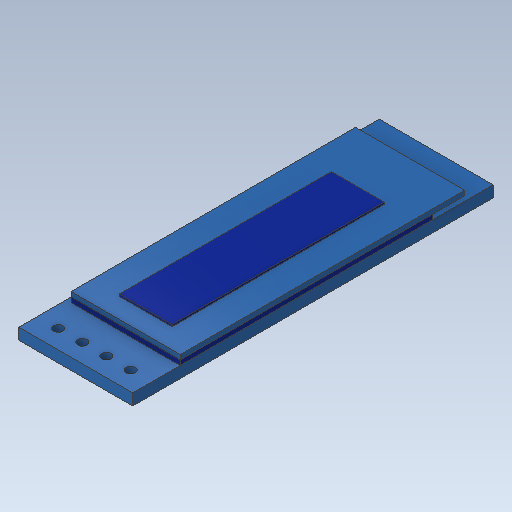
# Autodesk Inventor part: LED Screen 0.91 inch
Saved by Autodesk Inventor 2020.1 (Build 241239000, 239)
## iProperties
Created: 2019-07-16
Part Number: LED Screen 0.91 inch
Material: Generic
Document SubType Name: Modeling
Designer: Petar
Density: 1 g/cm^3
Appearance: Default
Mass: 0.805202 g
Surface Area: 16.0321 cm^2
Volume: 0.805202 cm^3
Author: Petar
Autodesk Inventor part; units mm, degrees
ref_plane "YZ Plane" through (0, 0, 0) normal (1, 0, 0) x (0, 1, 0)
ref_plane "XZ Plane" through (0, 0, 0) normal (0, 1, 0) x (-1, 0, 0)
sketch "Sketch1" plane through (0, 0, 0) normal (0, 1, 0) x (-1, 0, 0)
  line L0 (-6, 19) -> (6, 19)
  line L1 (6, 19) -> (6, -19)
  line L2 (6, -19) -> (-6, -19)
  line L3 (-6, -19) -> (-6, 19)
  line L4 (-6, 19) -> (6, -19) construction
  line L5 (6, 19) -> (-6, -19) construction
  line L6 (5.502, -16) -> (-5.998, -16)
  line L7 (5.502, 14) -> (5.502, -16)
  line L8 (0, 19) -> (0, -19) construction
  line L9 (5.503, 14.001) -> (-5.999, 14.001)
  line L10 (-5.999, 14.001) -> (-5.999, -12.599)
  line L11 (-5.999, -12.599) -> (5.503, -12.599)
  line L12 (3.541, 12.89) -> (-4.039, 12.89)
  line L13 (-4.039, 12.89) -> (-4.039, -11.49)
  line L14 (-4.039, -11.49) -> (3.541, -11.49)
  line L15 (3.541, -11.49) -> (3.541, 12.89)
  line L16 (2.541, 11.89) -> (-3.039, 11.89)
  line L17 (-3.039, 11.89) -> (-3.039, -10.49)
  line L18 (-3.039, -10.49) -> (2.541, -10.49)
  line L19 (2.541, -10.49) -> (2.541, 11.89)
  line L20 (-0.249, 12.89) -> (-0.249, -11.49) construction
  line L21 (3.541, 0.7) -> (-4.039, 0.7) construction
  circle A0 centre (-3.81, 17.04) radius 0.5
  circle A1 centre (-1.27, 17.04) radius 0.5
  circle A2 centre (1.27, 17.04) radius 0.5
  circle A3 centre (3.81, 17.04) radius 0.5
  line L22 (3.041, -13.8) -> (-3.539, -13.8)
  line L23 (-3.539, -13.8) -> (-3.539, -14.8)
  line L24 (-3.539, -14.8) -> (3.041, -14.8)
  line L25 (3.041, -14.8) -> (3.041, -13.8)
  line L26 (5.502, 14) -> (-5.998, 14)
  line L27 (5.503, -12.599) -> (5.503, 14.001)
  line L28 (-5.998, 14) -> (-5.998, -16)
  point P0 (0, 0)
  dimension "d0" = 12
  dimension "d1" = 38
  dimension "d2" = 3
  dimension "d3" = 30
  dimension "d5" = 26.6
  dimension "d6" = 7.58
  dimension "d7" = 24.38
  dimension "d8" = 5.58
  dimension "d9" = 22.38
  dimension "d10" = 1.96
  dimension "d11" = 7.51
  dimension "d13" = 2.19
  dimension "d14" = 1.96
  dimension "d15" = 1
  dimension "d18" = 2.54
  dimension "d27" = 1
  dimension "d28" = 1.2
  dimension "d32" = 0.001
  dimension "d33" = 0.001
  dimension "d34" = 0.001
  dimension "d35" = 11.5
  dimension "d36" = 0.001
  constraints: 58 end point, 11 parallel, 8 midpoint, 7 horizontal, 5 perpendicular, 4 centre point, 1 vertical, 10 other
  measures "d0" distance of L1.end L2.end
  measures "d1" distance of L0.end L1.end
  measures "d2" distance between parallel lines of L2 L6
  measures "d3" distance of L7.start L6.start
  measures "d5" distance of L10.end L9.end
  measures "d6" distance of L14.end L13.end
  measures "d7" distance of L13.end L12.end
  measures "d8" distance of L18.end L17.end
  measures "d9" distance of L17.end L16.end
  measures "d10" distance between parallel lines of L10 L13
  measures "d11" distance between parallel lines of L14 L2
  measures "d13" distance from line of L3 A0.centre
  measures "d14" distance from line of L0 A0.centre
  measures "d15" diameter of A0
  measures "d18" distance of A0.centre A1.centre
  measures "d27" distance of L23.end L22.end
  measures "d28" distance between parallel lines of L6 L24
  measures "d32" distance between parallel lines of L7 L27
  measures "d33" distance between parallel lines of L3 L10
  measures "d34" distance between parallel lines of L10 L28
  measures "d35" distance between parallel lines of L28 L7
  measures "d36" distance between parallel lines of L26 L9
extrude "Extrusion1" add sketch "Sketch1" against normal blind 1.2 contours L0 L1 L2 L3 L6 L7 L9 | L9 L7 L11 L3 | L11 L7 L6 L3 | L15 L14 L13 L12 | L19 L18 L17 L16 | L25 L24 L23 L22
extrude "Extrusion2" add sketch "Sketch1" along normal blind 0.5 contours L9 L7 L11 L3 | L15 L14 L13 L12 | L19 L18 L17 L16 | L25 L24 L23 L22
sketch "Sketch2" plane through (0, 0.5, 0) normal (0, 1, 0) x (1, 0, 0)
  line L0 (-5.502, -14) -> (-5.502, 16) projected
  line L1 (-5.502, 16) -> (5.998, 16) projected
  line L2 (-5.502, -14) -> (5.998, -14) projected
  line L3 (5.998, -14) -> (5.998, 16) projected
  line L4 (-3.541, -12.89) -> (4.039, -12.89) projected
  line L5 (-3.541, 11.49) -> (-3.541, -12.89) projected
  line L6 (4.039, -12.89) -> (4.039, 11.49) projected
  line L7 (4.039, 11.49) -> (-3.541, 11.49) projected
  point P0 (0, 0)
extrude "Extrusion3" add sketch "Sketch2" along normal blind 0.5 contours L0 L1 L3 L2 | L5 L7 L6 L4
sketch "Sketch3" plane through (0, 1, 0) normal (0, 1, 0) x (1, 0, 0)
  line L0 (-2.541, -11.89) -> (3.039, -11.89) projected
  line L1 (-2.541, 10.49) -> (-2.541, -11.89) projected
  line L2 (3.039, -11.89) -> (3.039, 10.49) projected
  line L3 (3.039, 10.49) -> (-2.541, 10.49) projected
  point P0 (0, 0)
extrude "Extrusion4" add sketch "Sketch3" along normal blind 0.2
extrude "Extrusion5" cut sketch "Sketch2" against normal blind 0.5 contours L5 L7 L6 L4
fillet "Fillet1" radius 1 4 edges at (-3.541, 0.25, 12.89) (4.039, 0.25, -11.49) (-3.541, 0.25, -11.49) (4.039, 0.25, 12.89)
sketch "Sketch4" plane through (0, -1.2, 0) normal (0, 1, 0) x (1, 0, 0)
  line L0 (2.785, -15.895) -> (2.585, -16.095)
  line L1 (2.585, -16.095) -> (2.585, -17.985)
  line L2 (2.585, -17.985) -> (2.785, -18.185)
  line L3 (2.785, -18.185) -> (4.835, -18.185)
  line L4 (4.835, -18.185) -> (5.035, -17.985)
  line L5 (5.035, -17.985) -> (5.035, -16.095)
  line L6 (5.035, -16.095) -> (4.835, -15.895)
  line L7 (4.835, -15.895) -> (2.785, -15.895)
  line L8 (3.81, -18.185) -> (3.81, -15.895) construction
  line L9 (2.585, -17.04) -> (5.035, -17.04) construction
  circle A0 centre (3.81, -17.04) radius 0.5 construction
  line L10 (3.51, -17.34) -> (4.11, -17.34)
  line L11 (4.11, -17.34) -> (4.11, -16.74)
  line L12 (4.11, -16.74) -> (3.51, -16.74)
  line L13 (3.51, -16.74) -> (3.51, -17.34)
  line L14 (3.51, -17.34) -> (4.11, -16.74) construction
  line L15 (4.11, -17.34) -> (3.51, -16.74) construction
  line L16 (6, -19) -> (-6, -19) construction
  line L17 (0.245, -15.895) -> (0.045, -16.095)
  line L18 (0.045, -16.095) -> (0.045, -17.985)
  line L19 (0.045, -17.985) -> (0.245, -18.185)
  line L20 (0.245, -18.185) -> (2.295, -18.185)
  line L21 (2.295, -18.185) -> (2.495, -17.985)
  line L22 (2.495, -17.985) -> (2.495, -16.095)
  line L23 (2.495, -16.095) -> (2.295, -15.895)
  line L24 (2.295, -15.895) -> (0.245, -15.895)
  line L25 (1.27, -18.185) -> (1.27, -15.895) construction
  line L26 (0.045, -17.04) -> (2.495, -17.04) construction
  circle A1 centre (1.27, -17.04) radius 0.5 construction
  line L27 (0.97, -17.34) -> (1.57, -17.34)
  line L28 (1.57, -17.34) -> (1.57, -16.74)
  line L29 (1.57, -16.74) -> (0.97, -16.74)
  line L30 (0.97, -16.74) -> (0.97, -17.34)
  line L31 (0.97, -17.34) -> (1.57, -16.74) construction
  line L32 (1.57, -17.34) -> (0.97, -16.74) construction
  line L33 (-2.295, -15.895) -> (-2.495, -16.095)
  line L34 (-2.495, -16.095) -> (-2.495, -17.985)
  line L35 (-2.495, -17.985) -> (-2.295, -18.185)
  line L36 (-2.295, -18.185) -> (-0.245, -18.185)
  line L37 (-0.245, -18.185) -> (-0.045, -17.985)
  line L38 (-0.045, -17.985) -> (-0.045, -16.095)
  line L39 (-0.045, -16.095) -> (-0.245, -15.895)
  line L40 (-0.245, -15.895) -> (-2.295, -15.895)
  line L41 (-1.27, -18.185) -> (-1.27, -15.895) construction
  line L42 (-2.495, -17.04) -> (-0.045, -17.04) construction
  circle A2 centre (-1.27, -17.04) radius 0.5 construction
  line L43 (-1.57, -17.34) -> (-0.97, -17.34)
  line L44 (-0.97, -17.34) -> (-0.97, -16.74)
  line L45 (-0.97, -16.74) -> (-1.57, -16.74)
  line L46 (-1.57, -16.74) -> (-1.57, -17.34)
  line L47 (-1.57, -17.34) -> (-0.97, -16.74) construction
  line L48 (-0.97, -17.34) -> (-1.57, -16.74) construction
  line L49 (-4.835, -15.895) -> (-5.035, -16.095)
  line L50 (-5.035, -16.095) -> (-5.035, -17.985)
  line L51 (-5.035, -17.985) -> (-4.835, -18.185)
  line L52 (-4.835, -18.185) -> (-2.785, -18.185)
  line L53 (-2.785, -18.185) -> (-2.585, -17.985)
  line L54 (-2.585, -17.985) -> (-2.585, -16.095)
  line L55 (-2.585, -16.095) -> (-2.785, -15.895)
  line L56 (-2.785, -15.895) -> (-4.835, -15.895)
  line L57 (-3.81, -18.185) -> (-3.81, -15.895) construction
  line L58 (-5.035, -17.04) -> (-2.585, -17.04) construction
  circle A3 centre (-3.81, -17.04) radius 0.5 construction
  line L59 (-4.11, -17.34) -> (-3.51, -17.34)
  line L60 (-3.51, -17.34) -> (-3.51, -16.74)
  line L61 (-3.51, -16.74) -> (-4.11, -16.74)
  line L62 (-4.11, -16.74) -> (-4.11, -17.34)
  line L63 (-4.11, -17.34) -> (-3.51, -16.74) construction
  line L64 (-3.51, -17.34) -> (-4.11, -16.74) construction
  circle A4 centre (-3.81, -17.04) radius 0.5 construction
  circle A5 centre (-1.27, -17.04) radius 0.5 construction
  circle A6 centre (1.27, -17.04) radius 0.5 construction
  point P0 (0, 0)
  point P1 (-1.27, -17.04)
  dimension "d43" = 2.05
  dimension "d46" = 1.89
  dimension "d47" = 0.2828
  dimension "d48" = 45
  dimension "d49" = 0.6
  dimension "d50" = 0.6
  dimension "d53" = 135
  dimension "d54" = 135
  dimension "d55" = 135
  dimension "d56" = 2.05
  dimension "d57" = 1.89
  dimension "d58" = 0.2828
  dimension "d59" = 45
  dimension "d60" = 0.6
  dimension "d61" = 0.6
  dimension "d62" = 135
  dimension "d63" = 135
  dimension "d64" = 135
  dimension "d65" = 2.05
  dimension "d66" = 1.89
  dimension "d67" = 0.2828
  dimension "d68" = 45
  dimension "d69" = 0.6
  dimension "d70" = 0.6
  dimension "d71" = 135
  dimension "d72" = 135
  dimension "d73" = 135
  dimension "d74" = 2.05
  dimension "d75" = 1.89
  dimension "d76" = 0.2828
  dimension "d77" = 45
  dimension "d78" = 0.6
  dimension "d79" = 0.6
  dimension "d80" = 135
  dimension "d81" = 135
  dimension "d82" = 135
  constraints: 128 end point, 31 midpoint, 20 equal length, 17 parallel, 8 perpendicular, 7 coincident, 4 horizontal, 3 centre point, 3 collinear
  measures "d43" distance of L6.end L0.start
  measures "d46" distance of L4.end L5.end
  measures "d47" distance of L5.end L6.end
  measures "d48" angle of L5 L6
  measures "d49" distance of L12.end L11.end
  measures "d50" distance of L11.end L10.end
  measures "d53" angle of L1 L0
  measures "d54" angle of L1 L2
  measures "d55" angle of L5 L4
  measures "d56" distance of L23.end L17.start
  measures "d57" distance of L22.start L22.end
  measures "d58" distance of L22.end L23.end
  measures "d59" angle of L22 L23
  measures "d60" distance of L29.end L29.start
  measures "d61" distance of L29.start L27.end
  measures "d62" angle of L18 L17
  measures "d63" angle of L18 L19
  measures "d64" angle of L22 L21
  measures "d65" distance of L39.end L33.start
  measures "d66" distance of L38.start L38.end
  measures "d67" distance of L38.end L39.end
  measures "d68" angle of L38 L39
  measures "d69" distance of L45.end L45.start
  measures "d70" distance of L45.start L43.end
  measures "d71" angle of L34 L33
  measures "d72" angle of L34 L35
  measures "d73" angle of L38 L37
  measures "d74" distance of L55.end L49.start
  measures "d75" distance of L54.start L54.end
  measures "d76" distance of L54.end L55.end
  measures "d77" angle of L54 L55
  measures "d78" distance of L61.end L61.start
  measures "d79" distance of L61.start L59.end
  measures "d80" angle of L50 L49
  measures "d81" angle of L50 L51
  measures "d82" angle of L54 L53
extrude "Extrusion6" [suppressed]
ref_plane "Work Plane2" through (0, 1.4, 0) normal (0, 1, 0) x (1, 0, 0)
sketch "Sketch5" plane through (0, 1.4, 0) normal (0, 1, 0) x (1, 0, 0)
  line L0 (4.11, -16.74) -> (4.11, -17.34) projected
  line L1 (4.11, -17.34) -> (3.51, -17.34) projected
  line L2 (3.51, -17.34) -> (3.51, -16.74) projected
  line L3 (3.51, -16.74) -> (4.11, -16.74) projected
  line L4 (1.57, -16.74) -> (1.57, -17.34) projected
  line L5 (0.97, -16.74) -> (1.57, -16.74) projected
  line L6 (1.57, -17.34) -> (0.97, -17.34) projected
  line L7 (0.97, -17.34) -> (0.97, -16.74) projected
  line L8 (-3.51, -16.74) -> (-3.51, -17.34) projected
  line L9 (-3.51, -17.34) -> (-4.11, -17.34) projected
  line L10 (-4.11, -17.34) -> (-4.11, -16.74) projected
  line L11 (-4.11, -16.74) -> (-3.51, -16.74) projected
  line L12 (-0.97, -16.74) -> (-0.97, -17.34) projected
  line L13 (-0.97, -17.34) -> (-1.57, -17.34) projected
  line L14 (-1.57, -17.34) -> (-1.57, -16.74) projected
  line L15 (-1.57, -16.74) -> (-0.97, -16.74) projected
  point P0 (0, 0)
  point P1 (4.11, 17.34)
  point P2 (4.11, 16.74)
  point P3 (3.51, 17.34)
  point P4 (3.51, 16.74)
  point P5 (1.57, 17.34)
  point P6 (1.57, 16.74)
  point P7 (0.97, 16.74)
  point P8 (0.97, 17.34)
  point P9 (-3.51, 17.34)
  point P10 (-3.51, 16.74)
  point P11 (-4.11, 17.34)
  point P12 (-4.11, 16.74)
  point P13 (-0.97, 17.34)
  point P14 (-0.97, 16.74)
  point P15 (-1.57, 17.34)
  point P16 (-1.57, 16.74)
  constraints: 8 other
extrude "Extrusion7" [suppressed]
body "Solid1"
body "Solid2"
